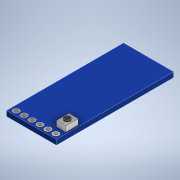
# Autodesk Inventor part: ZS-040
Saved by Autodesk Inventor 2021 (Build 250183000, 183)
## iProperties
Created: 2021-07-24
Part Number: ZS-040
Material: Generic
Document SubType Name: Modeling
Designer: ermoz
Density: 1 g/cm^3
Appearance: Default
Author: ermoz
Autodesk Inventor part; units mm, degrees
ref_plane "YZ Plane" through (0, 0, 0) normal (1, 0, 0) x (0, 1, 0)
ref_plane "XZ Plane" through (0, 0, 0) normal (0, 1, 0) x (-1, 0, 0)
ref_plane "XY Plane" through (0, 0, 0) normal (0, 0, 1) x (1, 0, 0)
sketch "Sketch1" plane through (0, 0, 0) normal (0, 1, 0) x (-1, 0, 0)
  line L0 (-8, -18.75) -> (8, -18.75)
  line L1 (8, -18.75) -> (8, 18.75)
  line L2 (8, 18.75) -> (-8, 18.75)
  line L3 (-8, 18.75) -> (-8, -18.75)
  line L4 (-8, -18.75) -> (8, 18.75) construction
  line L5 (8, -18.75) -> (-8, 18.75) construction
  point P0 (0, 0)
  dimension "d0" = 16
  dimension "d1" = 37.5
  constraints: 12 end point, 2 midpoint, 2 parallel, 1 horizontal, 1 perpendicular
  measures "d0" distance of L2.end L1.end
  measures "d1" distance of L1.end L0.end
extrude "Extrusion1" add sketch "Sketch1" along normal blind 1.6
sketch "Sketch2" plane through (0, 1.6, 0) normal (0, 1, 0) x (1, 0, 0)
  line L0 (4.5, -15.25) -> (7.5, -15.25)
  line L1 (7.5, -15.25) -> (7.5, -11.25)
  line L2 (7.5, -11.25) -> (4.5, -11.25)
  line L3 (4.5, -11.25) -> (4.5, -15.25)
  line L4 (8, -18.75) -> (8, 18.75) projected
  line L5 (-8, -18.75) -> (8, -18.75) projected
  point P0 (0, 0)
  dimension "d4" = 3
  dimension "d5" = 4
  dimension "d6" = 0.5
  dimension "d7" = 3.5
  constraints: 8 end point, 2 parallel, 1 horizontal, 1 perpendicular
  measures "d4" distance of L0.start L0.end
  measures "d5" distance of L0.end L1.end
  measures "d6" distance between parallel lines of L4 L1
  measures "d7" distance between parallel lines of L5 L0
extrude "Extrusion2" add sketch "Sketch2" along normal blind 1.75 separate body
sketch "Sketch3" plane through (0, 3.35, 0) normal (0, 1, 0) x (1, 0, 0)
  circle A0 centre (6, -13.25) radius 1
  line L0 (7.5, -11.25) -> (4.5, -11.25) projected
  line L1 (4.5, -11.25) -> (4.5, -15.25) projected
  point P0 (0, 0)
  point P1 (6, -11.25)
  point P2 (4.5, -13.25)
  dimension "d10" = 2
  constraints: 2 midpoint, 1 centre point, 1 horizontal alignment, 1 vertical alignment
  measures "d10" diameter of A0
extrude "Extrusion3" add sketch "Sketch3" along normal blind 0.5 separate body
sketch "Sketch4" plane through (0, 1.6, 0) normal (0, 1, 0) x (1, 0, 0)
  line L0 (0, 0) -> (0, -4.1131)
  circle A0 centre (1.27, -17.25) radius 0.5
  circle A1 centre (1.27, -17.25) radius 1
  circle A2 centre (3.81, -17.25) radius 0.5
  circle A3 centre (3.81, -17.25) radius 1
  circle A4 centre (6.35, -17.25) radius 0.5
  circle A5 centre (6.35, -17.25) radius 1
  line L1 (-8, -18.75) -> (8, -18.75) projected
  circle A6 centre (-1.27, -17.25) radius 0.5
  circle A7 centre (-1.27, -17.25) radius 1
  circle A8 centre (-3.81, -17.25) radius 0.5
  circle A9 centre (-3.81, -17.25) radius 1
  circle A10 centre (-6.35, -17.25) radius 0.5
  circle A11 centre (-6.35, -17.25) radius 1
  dimension "d13" = 2.54
  dimension "d14" = 2.54
  dimension "d15" = 1.27
  dimension "d16" = 1
  dimension "d17" = 2
  dimension "d20" = 1.5
  constraints: 12 centre point, 6 coincident, 6 symmetric about line, 4 equal radius, 2 end point, 2 horizontal alignment, 1 vertical, 6 other
  measures "d13" distance of A4.centre A2.centre
  measures "d14" distance of A0.centre A2.centre
  measures "d15" distance from line of L0 A0.centre
  measures "d16" diameter of A0
  measures "d17" diameter of A1
  measures "d20" distance from line of L1 A0.centre
extrude "Extrusion4" cut sketch "Sketch4" against normal through all contours A0 | A1 | A2 | A3 | A4 | A5 | A6 | A7 | A8 | A9 | A10 | A11 bodies 1
extrude "Extrusion5" add sketch "Sketch4" against normal up to surface (1.6 mm away) separate body
body "Solid1"
body "Solid2"
body "Solid3"
body "Solid4"
